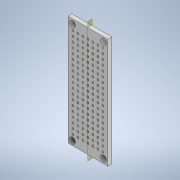
# Autodesk Inventor part: KLEPKNOP2
Saved by Autodesk Inventor 2020 (Build 240168000, 168)
## iProperties
Created: 2020-06-10
Part Number: KLEPKNOP2
Material: Generic
Document SubType Name: Modeling
Designer: Gebruiker
Density: 1 g/cm^3
Appearance: Default
Author: Gebruiker
Autodesk Inventor part; units mm, degrees
ref_plane "YZ Plane" through (0, 0, 0) normal (1, 0, 0) x (0, 1, 0)
ref_plane "XZ Plane" through (0, 0, 0) normal (0, 1, 0) x (-1, 0, 0)
ref_plane "XY Plane" through (0, 0, 0) normal (0, 0, 1) x (1, 0, 0)
sketch "Sketch1" plane through (0, 0, 0) normal (0, 0, 1) x (1, 0, 0)
  line L0 (-10, 27.5) -> (10, 27.5)
  line L1 (10, 27.5) -> (10, -27.5)
  line L2 (10, -27.5) -> (-10, -27.5)
  line L3 (-10, -27.5) -> (-10, 27.5)
  line L4 (-10, 27.5) -> (10, -27.5) construction
  line L5 (10, 27.5) -> (-10, -27.5) construction
  line L6 (-10, 22.5) -> (10, 22.5) construction
  circle A0 centre (-7.5, 22.5) radius 0.5
  circle A1 centre (-7.5, 20) radius 0.5
  circle A2 centre (-7.5, 17.5) radius 0.5
  circle A3 centre (-7.5, 15) radius 0.5
  circle A4 centre (-7.5, 12.5) radius 0.5
  circle A5 centre (-7.5, 10) radius 0.5
  circle A6 centre (-7.5, 7.5) radius 0.5
  circle A7 centre (-7.5, 5) radius 0.5
  circle A8 centre (-7.5, 2.5) radius 0.5
  circle A9 centre (-7.5, 0) radius 0.5
  circle A10 centre (-7.5, -2.5) radius 0.5
  circle A11 centre (-7.5, -5) radius 0.5
  circle A12 centre (-7.5, -7.5) radius 0.5
  circle A13 centre (-7.5, -10) radius 0.5
  circle A14 centre (-7.5, -12.5) radius 0.5
  circle A15 centre (-7.5, -15) radius 0.5
  circle A16 centre (-7.5, -17.5) radius 0.5
  circle A17 centre (-7.5, -20) radius 0.5
  circle A18 centre (-7.5, -22.5) radius 0.5
  circle A19 centre (-5, 22.5) radius 0.5
  circle A20 centre (-5, 20) radius 0.5
  circle A21 centre (-5, 17.5) radius 0.5
  circle A22 centre (-5, 15) radius 0.5
  circle A23 centre (-5, 12.5) radius 0.5
  circle A24 centre (-5, 10) radius 0.5
  circle A25 centre (-5, 7.5) radius 0.5
  circle A26 centre (-5, 5) radius 0.5
  circle A27 centre (-5, 2.5) radius 0.5
  circle A28 centre (-5, 0) radius 0.5
  circle A29 centre (-5, -2.5) radius 0.5
  circle A30 centre (-5, -5) radius 0.5
  circle A31 centre (-5, -7.5) radius 0.5
  circle A32 centre (-5, -10) radius 0.5
  circle A33 centre (-5, -12.5) radius 0.5
  circle A34 centre (-5, -15) radius 0.5
  circle A35 centre (-5, -17.5) radius 0.5
  circle A36 centre (-5, -20) radius 0.5
  circle A37 centre (-5, -22.5) radius 0.5
  circle A38 centre (-2.5, 22.5) radius 0.5
  circle A39 centre (-2.5, 20) radius 0.5
  circle A40 centre (-2.5, 17.5) radius 0.5
  circle A41 centre (-2.5, 15) radius 0.5
  circle A42 centre (-2.5, 12.5) radius 0.5
  circle A43 centre (-2.5, 10) radius 0.5
  circle A44 centre (-2.5, 7.5) radius 0.5
  circle A45 centre (-2.5, 5) radius 0.5
  circle A46 centre (-2.5, 2.5) radius 0.5
  circle A47 centre (-2.5, 0) radius 0.5
  circle A48 centre (-2.5, -2.5) radius 0.5
  circle A49 centre (-2.5, -5) radius 0.5
  circle A50 centre (-2.5, -7.5) radius 0.5
  circle A51 centre (-2.5, -10) radius 0.5
  circle A52 centre (-2.5, -12.5) radius 0.5
  circle A53 centre (-2.5, -15) radius 0.5
  circle A54 centre (-2.5, -17.5) radius 0.5
  circle A55 centre (-2.5, -20) radius 0.5
  circle A56 centre (-2.5, -22.5) radius 0.5
  circle A57 centre (0, 22.5) radius 0.5
  circle A58 centre (0, 20) radius 0.5
  circle A59 centre (0, 17.5) radius 0.5
  circle A60 centre (0, 15) radius 0.5
  circle A61 centre (0, 12.5) radius 0.5
  circle A62 centre (0, 10) radius 0.5
  circle A63 centre (0, 7.5) radius 0.5
  circle A64 centre (0, 5) radius 0.5
  circle A65 centre (0, 2.5) radius 0.5
  circle A66 centre (0, 0) radius 0.5
  circle A67 centre (0, -2.5) radius 0.5
  circle A68 centre (0, -5) radius 0.5
  circle A69 centre (0, -7.5) radius 0.5
  circle A70 centre (0, -10) radius 0.5
  circle A71 centre (0, -12.5) radius 0.5
  circle A72 centre (0, -15) radius 0.5
  circle A73 centre (0, -17.5) radius 0.5
  circle A74 centre (0, -20) radius 0.5
  circle A75 centre (0, -22.5) radius 0.5
  circle A76 centre (2.5, 22.5) radius 0.5
  circle A77 centre (2.5, 20) radius 0.5
  circle A78 centre (2.5, 17.5) radius 0.5
  circle A79 centre (2.5, 15) radius 0.5
  circle A80 centre (2.5, 12.5) radius 0.5
  circle A81 centre (2.5, 10) radius 0.5
  circle A82 centre (2.5, 7.5) radius 0.5
  circle A83 centre (2.5, 5) radius 0.5
  circle A84 centre (2.5, 2.5) radius 0.5
  circle A85 centre (2.5, 0) radius 0.5
  circle A86 centre (2.5, -2.5) radius 0.5
  circle A87 centre (2.5, -5) radius 0.5
  circle A88 centre (2.5, -7.5) radius 0.5
  circle A89 centre (2.5, -10) radius 0.5
  circle A90 centre (2.5, -12.5) radius 0.5
  circle A91 centre (2.5, -15) radius 0.5
  circle A92 centre (2.5, -17.5) radius 0.5
  circle A93 centre (2.5, -20) radius 0.5
  circle A94 centre (2.5, -22.5) radius 0.5
  circle A95 centre (5, 22.5) radius 0.5
  circle A96 centre (5, 20) radius 0.5
  circle A97 centre (5, 17.5) radius 0.5
  circle A98 centre (5, 15) radius 0.5
  circle A99 centre (5, 12.5) radius 0.5
  circle A100 centre (5, 10) radius 0.5
  circle A101 centre (5, 7.5) radius 0.5
  circle A102 centre (5, 5) radius 0.5
  circle A103 centre (5, 2.5) radius 0.5
  circle A104 centre (5, 0) radius 0.5
  circle A105 centre (5, -2.5) radius 0.5
  circle A106 centre (5, -5) radius 0.5
  circle A107 centre (5, -7.5) radius 0.5
  circle A108 centre (5, -10) radius 0.5
  circle A109 centre (5, -12.5) radius 0.5
  circle A110 centre (5, -15) radius 0.5
  circle A111 centre (5, -17.5) radius 0.5
  circle A112 centre (5, -20) radius 0.5
  circle A113 centre (5, -22.5) radius 0.5
  circle A114 centre (7.5, 22.5) radius 0.5
  circle A115 centre (7.5, 20) radius 0.5
  circle A116 centre (7.5, 17.5) radius 0.5
  circle A117 centre (7.5, 15) radius 0.5
  circle A118 centre (7.5, 12.5) radius 0.5
  circle A119 centre (7.5, 10) radius 0.5
  circle A120 centre (7.5, 7.5) radius 0.5
  circle A121 centre (7.5, 5) radius 0.5
  circle A122 centre (7.5, 2.5) radius 0.5
  circle A123 centre (7.5, 0) radius 0.5
  circle A124 centre (7.5, -2.5) radius 0.5
  circle A125 centre (7.5, -5) radius 0.5
  circle A126 centre (7.5, -7.5) radius 0.5
  circle A127 centre (7.5, -10) radius 0.5
  circle A128 centre (7.5, -12.5) radius 0.5
  circle A129 centre (7.5, -15) radius 0.5
  circle A130 centre (7.5, -17.5) radius 0.5
  circle A131 centre (7.5, -20) radius 0.5
  circle A132 centre (7.5, -22.5) radius 0.5
  point P0 (0, 0)
  dimension "d0" = 20
  dimension "d1" = 55
  dimension "d2" = 1
  dimension "d3" = 2.5
  dimension "d4" = 5
  dimension "d7" = 2.5
  dimension "d10" = 2.5
  constraints: 133 centre point, 14 end point, 3 point on line, 2 horizontal, 2 midpoint, 2 parallel, 2 perpendicular, 1 vertical, 264 other
  measures "d0" distance of L1.end L2.end
  measures "d1" distance of L0.end L1.end
  measures "d2" diameter of A0
  measures "d3" distance from line of L3 A0.centre
  measures "d4" distance from line of A0.centre L0
  measures "d7" distance of A0.centre A1.centre
  measures "d10" distance of A0.centre A19.centre
extrude "Extrusion1" add sketch "Sketch1" against normal blind 2
sketch "Sketch2" plane through (0, 0, 0) normal (0, 0, 1) x (1, 0, 0)
  circle A0 centre (-7.7572, 25.2572) radius 1.5
  line L0 (-10, 27.5) -> (10, 27.5) projected
  line L1 (-10, 27.5) -> (-10, -27.5) projected
  line L2 (-7.7572, 25.2572) -> (-7.7572, 27.5) construction
  line L3 (-7.7572, 25.2572) -> (-10, 25.2572) construction
  line L4 (-10, -27.5) -> (-10, 27.5) construction
  point P0 (0, 0)
  dimension "d15" = 3
  dimension "d18" = 2.2428
  constraints: 4 end point, 2 perpendicular, 2 point on line, 1 centre point, 1 vertical
  measures "d15" diameter of A0
  measures "d18" distance of L3.end L2.start
extrude "Extrusion2" cut sketch "Sketch2" against normal blind 2
mirror "Mirror1" about plane through (0, 0, 0) normal (1, 0, 0) of "Extrusion2"
mirror "Mirror2" about plane through (0, 0, 0) normal (0, 1, 0) of "Extrusion2", "Mirror1"
ref_plane "Work Plane1" through (0, 0, 0) normal (1, 0, 0) x (0, 1, 0)
ref_plane "Work Plane2" through (0, 0, 0) normal (-1, 0, 0) x (0, -1, 0)
ref_plane "Work Plane3" through (0, 0, 0) normal (-1, 0, 0) x (0, -1, 0)
body "Solid1"
